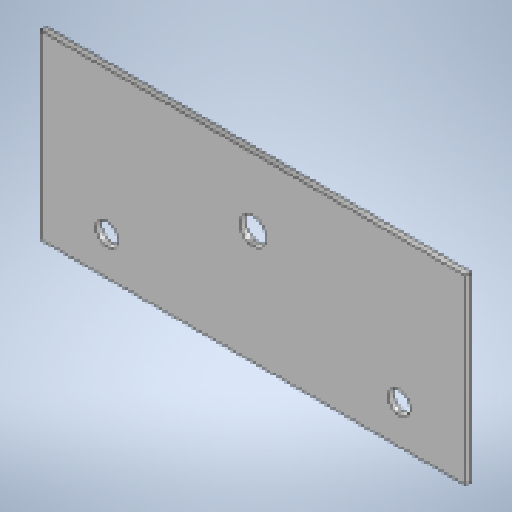
# Autodesk Inventor part: DMF 01 15 drum sheet 1
Saved by Autodesk Inventor 2026.2 (Build 302298010, 298A)
## iProperties
Created: 2024-04-28
Part Number: DMF 01 15 drum sheet 1
Material: Stainless Steel AISI 304
Document SubType Name: Sheet Metal
Designer: admin
Stock Number: Барабан_Лист_Правый_Борт
Density: 8 g/cm^3
Flat Pattern Width: 9 cm
Flat Pattern Length: 21.11 cm
Flat Pattern Area: 189.99 cm^2
Sheet Metal Rule: Default
Sheet Metal Width: 90,000 mm
Sheet Metal Length: 211,100 mm
Sheet Metal Area: 18999,000 mm^2
Appearance: Chrome - Satin
Author: pokla
Autodesk Inventor part; units mm, degrees
ref_plane "YZ Plane" through (0, 0, 0) normal (1, 0, 0) x (0, 1, 0)
ref_plane "XZ Plane" through (0, 0, 0) normal (0, 1, 0) x (-1, 0, 0)
ref_plane "XY Plane" through (0, 0, 0) normal (0, 0, 1) x (1, 0, 0)
sketch "Sketch15" plane through (0, 0, 0) normal (0, 0, 1) x (1, 0, 0)
  line L0 (-105.55, 45) -> (105.55, 45)
  line L1 (105.55, 45) -> (105.55, -45)
  line L2 (105.55, -45) -> (-105.55, -45)
  line L3 (-105.55, -45) -> (-105.55, 45)
  line L4 (-105.55, 45) -> (105.55, -45) construction
  line L5 (105.55, 45) -> (-105.55, -45) construction
  circle A0 centre (0, 11.5) radius 6.5
  circle A1 centre (72.5, -26) radius 5.5
  circle A2 centre (-72.5, -26) radius 5.5
  line L6 (0, 0) -> (0, -45) construction
  dimension "d173" = 211.1
  dimension "d174" = 90
  dimension "d176" = 13
  dimension "d177" = 11
  dimension "d178" = 11.5
  dimension "d179" = 26
  dimension "d180" = 145
  measures "d173" distance of L1.end L2.end
  measures "d174" distance of L0.end L1.end
  measures "d176" diameter of A0
  measures "d177" diameter of A1
  measures "d178" distance of L6.start A0.centre
  measures "d179" vertical distance of L6.start A1.centre
  measures "d180" distance of A2.centre A1.centre
extrude "Plate10" add sketch "Sketch15" along normal blind 3
equation "\"BendRadius\" = Thickness"
equation "\"BendReliefWidth\" = Thickness"
equation "\"BendReliefDepth\" = 0.5 * Thickness"
equation "\"CornerReliefSize\" = 4 * Thickness"
equation "\"MinimumRemnant\" = 2 * Thickness"
equation "\"TransitionRadius\" = BendRadius"
equation "\"JacobiRadiusSize\" = BendRadius"
equation "\"GapSize\" = Thickness"
equation "\"Thickness\" = 3"
body "Solid3"
